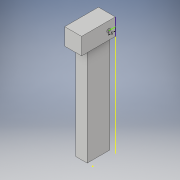
# Autodesk Inventor part: detector curvament fil
Saved by Autodesk Inventor 2019 (Build 230136000, 136)
## iProperties
Created: 2018-08-06
Part Number: detector curvament fil
Material: Genérico
Document SubType Name: Modeling
Designer: Albert Garangou Culebras
Density: 1 g/cm^3
Appearance: Valor por defecto
Mass: 54.1896 g
Surface Area: 120.446 cm^2
Volume: 54.1896 cm^3
Author: Albert Garangou Culebras
Title: suport detector curvament fil
Comments: Falta fer una possible guia per amagar el cable (dins la paret o a fora).
Autodesk Inventor part; units mm, degrees
ref_plane "YZ Plane" through (0, 0, 0) normal (1, 0, 0) x (0, 1, 0)
ref_plane "XZ Plane" through (0, 0, 0) normal (0, 1, 0) x (-1, 0, 0)
ref_plane "XY Plane" through (0, 0, 0) normal (0, 0, 1) x (1, 0, 0)
sketch "base" plane through (0, 0, 0) normal (0, 1, 0) x (-1, 0, 0)
  line L0 (0, 0) -> (0, -20)
  line L1 (0, -20) -> (10, -20)
  line L2 (10, -20) -> (10, 0)
  line L3 (10, 0) -> (0, 0)
  dimension "d186" = 20
  dimension "d187" = 10
  constraints: 8 end point, 3 perpendicular, 1 vertical
  measures "d186" distance of L0.start L0.end
  measures "d187" distance of L0.end L1.end
extrude "Extrusión29" add sketch "base" along normal blind 90
sketch "Boceto41" plane through (0, 90, 0) normal (0, 1, 0) x (1, 0, 0)
  line L0 (0, 20) -> (5, 20)
  line L1 (5, 20) -> (5, 0)
  line L2 (-10, 0) -> (0, 0) projected
  line L3 (5, 0) -> (-10, 0)
  line L4 (-10, 0) -> (-10, 20)
  line L5 (-10, 20) -> (5, 20)
  dimension "d190" = 5
  constraints: 10 end point, 2 collinear, 2 perpendicular, 1 horizontal, 1 point on line
  measures "d190" distance of L0.start L0.end
extrude "Extrusión30" add sketch "Boceto41" along normal blind 15
sketch "Boceto42" plane through (-10, 0, 0) normal (0, 0, 1) x (1, 0, 0)
  line L0 (15, 90) -> (10, 90) projected
  line L1 (15, 90) -> (0, 90)
  line L2 (0, 0) -> (0, 105) projected
  line L3 (0, 90) -> (0, 105)
  line L4 (0, 105) -> (15, 105) projected
  line L5 (0, 105) -> (15, 105)
  line L6 (15, 105) -> (15, 90)
  point P0 (10, 0)
  constraints: 8 end point, 2 perpendicular, 1 collinear, 1 horizontal
extrude "Extrusión31" add sketch "Boceto42" along normal blind 10
sketch "Boceto45" plane through (5, 90, -20) normal (1, 0, 0) x (0, 0, -1)
  line L0 (0, -90) -> (0, 15) projected
  line L1 (0, 0) -> (0, 15)
  line L2 (0, 7.5) -> (-6, 7.5)
  point P0 (-20, -90)
  dimension "d200" = 6
  constraints: 4 end point, 1 collinear, 1 horizontal, 1 midpoint
  measures "d200" distance of L2.start L2.end
hole "Agujero1" at (5, 97.5, -14) direction (-1, 0, 0) diameter 3.2 end through all
sketch "Boceto51" plane through (-10, 0, -20) normal (-1, 0, 0) x (0, 0, 1)
  circle A0 centre (6, 97.5) radius 1.6 projected
  circle A1 centre (6, 97.5) radius 1.6
  point P0 (20, 0)
  constraints: 1 centre point, 1 coincident
hole "Agujero2" at (-10, 97.5, -14) direction (1, 0, 0) diameter 3.2 depth 30 counterbore diameter 10 counterbore depth 5
